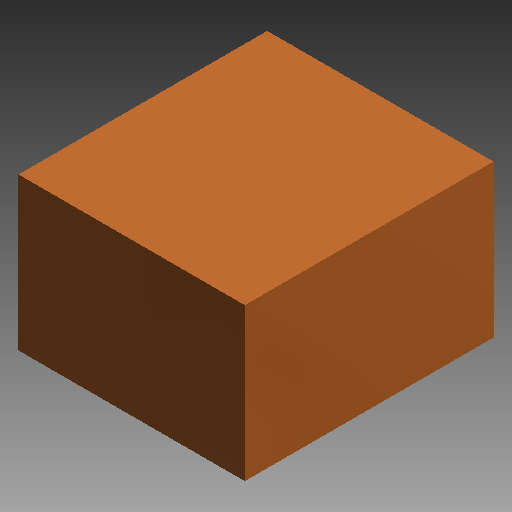
# Autodesk Inventor part: PINHD-2X3
Saved by Autodesk Inventor 2018.2 (Build 222227000, 227)
## iProperties
Part Number: PINHD-2X3
Material: Generic
Document SubType Name: Modeling
Designer: autocad
Appearance: 2X03, PINHD-2X3
Author: autocad
Autodesk Inventor part; units mm, degrees
ref_plane "YZ Plane" through (0, 0, 0) normal (1, 0, 0) x (0, 1, 0)
ref_plane "XZ Plane" through (0, 0, 0) normal (0, 1, 0) x (-1, 0, 0)
ref_plane "XY Plane" through (0, 0, 0) normal (0, 0, 1) x (1, 0, 0)
sketch "2X03, PINHD-2X3_283" plane through (0, 0, 0) normal (0, 0, 1) x (1, 0, 0)
  line L0 (3.8862, -2.6162) -> (-3.8862, -2.6162)
  line L1 (-3.8862, -2.6162) -> (-3.8862, 2.6162)
  line L2 (-3.8862, 2.6162) -> (3.8862, 2.6162)
  line L3 (3.8862, 2.6162) -> (3.8862, -2.6162)
  constraints: 8 end point
extrude "Extrusion1" add sketch "2X03, PINHD-2X3_283" along normal blind 8.54
body "Solid1"
